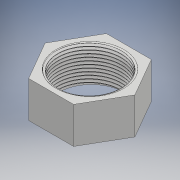
# Autodesk Inventor part: Tuerca
Saved by Autodesk Inventor 2018 (Build 220112000, 112)
## iProperties
Created: 2019-11-18
Part Number: Tuerca
Material: Generic
Document SubType Name: Modeling
Designer: Marie
Density: 1 g/cm^3
Appearance: Default
Author: Marie
Autodesk Inventor part; units mm, degrees
ref_plane "YZ Plane" through (0, 0, 0) normal (1, 0, 0) x (0, 1, 0)
ref_plane "XZ Plane" through (0, 0, 0) normal (0, 1, 0) x (-1, 0, 0)
ref_plane "XY Plane" through (0, 0, 0) normal (0, 0, 1) x (1, 0, 0)
sketch "Sketch1" plane through (0, 0, 0) normal (0, 0, 1) x (1, 0, 0)
  circle A0 centre (0, 0) radius 32.5
  line L0 (43.1593, 0) -> (21.5796, -37.377)
  line L1 (21.5796, -37.377) -> (-21.5796, -37.377)
  line L2 (-21.5796, -37.377) -> (-43.1593, 0)
  line L3 (-43.1593, 0) -> (-21.5796, 37.377)
  line L4 (-21.5796, 37.377) -> (21.5796, 37.377)
  line L5 (21.5796, 37.377) -> (43.1593, 0)
  dimension "d0" = 65
  constraints: 12 end point, 2 coincident, 1 centre point, 13 other
  measures "d0" diameter of A0
extrude "Extrusion1" add sketch "Sketch1" along normal blind 35
thread "Thread3" size "M65x3" class "6H" standard "ANSI Metric M Profile" full length
sketch "Sketch7" plane through (0, 0, 35) normal (-1, 0, 0) x (0, 1, 0)
  line L0 (32.5, 0) -> (32.5, 35)
  line L1 (32.5, 35) -> (30.2756, 35)
  line L2 (30.2756, 35) -> (30.2756, 0)
  line L3 (30.2756, 0) -> (32.5, 0)
  line L4 (0, -10.9256) -> (0, 42.6543) projected
  constraints: 8 end point
revolve "Revolution3" add sketch "Sketch7" angle 360 about axis through (0, 0, 35) along (0, 0, -1) separate body
sketch "Sketch6" plane through (0, 32.5, 35) normal (1, 0, 0) x (0, 0, -1)
  line L0 (-1.7501, -0.1519) -> (-1.5001, -0.1519) construction
  line L1 (0.2499, -2.0728) -> (-0.0001, -2.5531) construction
  line L2 (-3.0001, -2.5531) -> (-3.2501, -2.0728) construction
  line L3 (-1.2501, -0.1519) -> (-1.5001, 0.3284) construction
  line L4 (-1.5001, 0.3284) -> (-1.7501, -0.1519) construction
  line L5 (-3.0001, -2.5531) -> (-2.7501, -2.0728) construction
  line L6 (-1.2501, -0.1519) -> (-0.2501, -2.0728)
  line L7 (-3.2501, -2.0728) -> (-2.7501, -2.0728) construction
  arc A0 (-3.2501, -2.0728) -> (-3.0001, -2.2246) centre (-3.0001, -1.9427) ccw construction
  line L8 (0.2499, -2.0728) -> (-0.2501, -2.0728) construction
  line L9 (-3.0001, -2.5531) -> (-3.0001, -2.0728) construction
  line L10 (-0.0001, -2.5531) -> (-0.0001, -2.0728) construction
  line L11 (-1.5001, 0.3284) -> (-1.5001, -0.0002) construction
  line L12 (-3.0001, -2.2246) -> (-0.0001, -2.2246)
  arc A1 (-3.0001, -2.2246) -> (-2.7501, -2.0728) centre (-3.0001, -1.9427) ccw
  line L13 (-0.2501, -2.0728) -> (-0.0001, -2.5531) construction
  line L14 (-2.7501, -2.0728) -> (-1.7501, -0.1519)
  line L15 (-0.0001, -0.0002) -> (-0.0001, 0.0177)
  line L16 (-0.0001, 0.0177) -> (-0.0001, -0.0002)
  line L17 (-0.0001, -0.0002) -> (0.0334, -0.0002)
  arc A2 (-0.2501, -2.0728) -> (-0.0001, -2.2246) centre (-0.0001, -1.9427) ccw
  arc A3 (-0.0001, -2.2246) -> (0.2499, -2.0728) centre (-0.0001, -1.9427) ccw construction
  arc A4 (-1.5001, -0.0002) -> (-1.7501, -0.1519) centre (-1.5001, -0.282) ccw
  arc A5 (-1.2501, -0.1519) -> (-1.5001, -0.0002) centre (-1.5001, -0.282) ccw
  line L18 (-1.5001, -0.0002) -> (-1.5001, -0.1519) construction
  line L19 (-1.5001, -0.1519) -> (-1.2501, -0.1519) construction
  dimension "d45" = 55
  dimension "d46" = 0.4803
  dimension "d47" = 0.4803
  dimension "Sketch6_ThreadOffset" = 0
  dimension "Sketch6_MajorRadius" = 2.2244
  dimension "d50" = 3
  dimension "Sketch6_MinorRadius" = 0
  constraints: 40 end point, 12 point on circle, 10 parallel, 8 tangent, 6 centre point, 6 collinear, 2 midpoint, 2 point on line, 1 horizontal, 1 perpendicular, 3 other
  measures "d45" angle of L6 L14
  measures "d46" distance of L3.end L0.end
  measures "d47" distance of L1.end L10.end
  measures "Sketch6_ThreadOffset" distance between parallel lines of L15 L10
  measures "Sketch6_MajorRadius" distance from line of L12 L15.start
  measures "d50" distance from line of L1.end L9
  measures "Sketch6_MinorRadius" distance edge to line of A5 L17
coil "Coil3" sketch "Sketch6" operation cut axis through (0, 0, 35) along (0, 0, -1) pitch 3.003 turns 13.653014 hand right bodies 2
equation "\"d45\" = d52"
equation "\"d46\" = 0.160083 * Sketch6_Pitch"
equation "\"d47\" = 0.160083 * Sketch6_Pitch"
equation "\"d50\" = Sketch6_Pitch"
equation "\"d12\" = 55deg"
equation "\"Sketch2_Pitch\" = 3"
equation "\"d32\" = 55deg"
equation "\"Sketch4_Pitch\" = 3"
equation "\"d52\" = 55deg"
equation "\"Sketch6_Pitch\" = 3"
body "Solid1"
body "Solid4"
